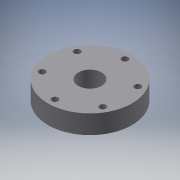
# Autodesk Inventor part: spacer
Saved by Autodesk Inventor 2016 (Build 200138000, 138)
## iProperties
Created: 2016-01-17
Part Number: spacer
Material: Generic
Document SubType Name: Modeling
Designer: gus
Density: 1 g/cm^3
Appearance: Default
Author: gus
Autodesk Inventor part; units mm, degrees
ref_plane "YZ Plane" through (0, 0, 0) normal (1, 0, 0) x (0, 1, 0)
ref_plane "XZ Plane" through (0, 0, 0) normal (0, 1, 0) x (-1, 0, 0)
ref_plane "XY Plane" through (0, 0, 0) normal (0, 0, 1) x (1, 0, 0)
sketch "Sketch1" plane through (0, 0, 0) normal (0, 1, 0) x (-1, 0, 0)
  circle A0 centre (0, 0) radius 23.8125 construction
  circle A1 centre (0, 23.8125) radius 2.159
  line L0 (0, 0) -> (0, 23.8125) construction
  line L1 (0, 23.8125) -> (20.6222, 11.9062) construction
  line L2 (20.6222, 11.9062) -> (20.6222, -11.9062) construction
  line L3 (20.6222, -11.9062) -> (0, -23.8125) construction
  line L4 (0, -23.8125) -> (-20.6222, -11.9063) construction
  line L5 (-20.6222, -11.9063) -> (-20.6222, 11.9062) construction
  line L6 (-20.6222, 11.9062) -> (0, 23.8125) construction
  circle A2 centre (-20.6222, 11.9062) radius 2.159
  circle A3 centre (-20.6222, -11.9063) radius 2.159
  circle A4 centre (0, -23.8125) radius 2.159
  circle A5 centre (20.6222, -11.9062) radius 2.159
  circle A6 centre (20.6222, 11.9062) radius 2.159
  circle A7 centre (0, 0) radius 28.575
  circle A8 centre (0, 0) radius 7.9375
  dimension "d0" = 47.625
  dimension "d1" = 4.318
  dimension "d2" = 4.318
  dimension "d3" = 4.318
  dimension "d4" = 4.318
  dimension "d5" = 4.318
  dimension "d6" = 4.318
  dimension "d7" = 57.15
  dimension "d10" = 15.875
  constraints: 14 end point, 9 coincident, 8 centre point, 1 vertical, 1 vertical alignment, 15 other
  measures "d1" diameter of A1
  measures "d2" diameter of A2
  measures "d3" diameter of A3
  measures "d4" diameter of A4
  measures "d5" diameter of A5
  measures "d6" diameter of A6
  measures "d7" diameter of A7
  measures "d10" diameter of A8
extrude "Extrusion2" add sketch "Sketch1" along normal blind 12.7762
body "Solid2"
